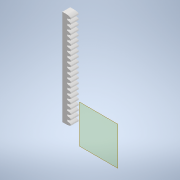
# Autodesk Inventor part: Zahnstange
Saved by Autodesk Inventor 2021 (Build 250183000, 183)
## iProperties
Created: 2021-01-13
Part Number: Zahnstange
Material: Generisch
Document SubType Name: Modeling
Designer: LETPJG
Density: 1 g/cm^3
Appearance: Vorgabe
Author: LETPJG
Autodesk Inventor part; units mm, degrees
ref_plane "YZ Plane" through (0, 0, 0) normal (1, 0, 0) x (0, 1, 0)
ref_plane "XZ Plane" through (0, 0, 0) normal (0, 1, 0) x (-1, 0, 0)
ref_plane "XY Plane" through (0, 0, 0) normal (0, 0, 1) x (1, 0, 0)
ref_plane "Arbeitsebene1" through (0, 0, -5) normal (0, 0, -1) x (-1, 0, 0)
sketch "Skizze1" plane through (0, 0, -5) normal (0, 0, -1) x (-1, 0, 0)
  arc A0 (8.6893, -1.0285) -> (10.9915, -0.4319) centre (7.7825, 7.211) ccw
  arc A1 (10.9915, -0.4319) -> (10.9915, 0.4319) centre (0, 0) ccw
  arc A2 (10.9915, 0.4319) -> (8.6893, 1.0285) centre (7.7825, -7.211) ccw
  line L0 (8.6893, -1.0285) -> (8.6893, 1.0285) construction
  arc A3 (12.6615, 1.2584) -> (14.9637, 0.6618) centre (15.8705, 8.9013) ccw
  arc A4 (12.6615, 2.1221) -> (12.6615, 1.2584) centre (23.6531, 1.6903) ccw
  arc A5 (14.9637, 2.7187) -> (12.6615, 2.1221) centre (15.8705, -5.5208) ccw
  arc A6 (8.6893, 1.0285) -> (8.5819, 1.707) centre (0, 0) ccw construction
  arc A7 (8.6893, 1.0285) -> (8.5819, 1.707) centre (0, 0) ccw construction
  arc A8 (8.6893, 1.0285) -> (8.5819, 1.707) centre (0, 0) ccw construction
  arc A9 (8.6893, 1.0285) -> (8.5819, 1.707) centre (0, 0) ccw construction
  arc A10 (8.6893, 1.0285) -> (8.5819, 1.707) centre (0, 0) ccw construction
  arc A11 (12.6615, 4.1794) -> (14.9637, 3.5828) centre (15.8705, 11.8223) ccw
  arc A12 (12.6615, 5.0431) -> (12.6615, 4.1794) centre (23.6531, 4.6113) ccw
  arc A13 (14.9637, 5.6397) -> (12.6615, 5.0431) centre (15.8705, -2.5998) ccw
  arc A14 (12.6615, 7.1004) -> (14.9637, 6.5038) centre (15.8705, 14.7433) ccw
  arc A15 (12.6615, 7.9641) -> (12.6615, 7.1004) centre (23.6531, 7.5323) ccw
  arc A16 (14.9637, 8.5607) -> (12.6615, 7.9641) centre (15.8705, 0.3212) ccw
  arc A17 (12.6615, 10.0214) -> (14.9637, 9.4248) centre (15.8705, 17.6643) ccw
  arc A18 (12.6615, 10.8851) -> (12.6615, 10.0214) centre (23.6531, 10.4533) ccw
  arc A19 (14.9637, 11.4817) -> (12.6615, 10.8851) centre (15.8705, 3.2422) ccw
  arc A20 (12.6615, 12.9424) -> (14.9637, 12.3458) centre (15.8705, 20.5853) ccw
  arc A21 (12.6615, 13.8061) -> (12.6615, 12.9424) centre (23.6531, 13.3743) ccw
  arc A22 (14.9637, 14.4027) -> (12.6615, 13.8061) centre (15.8705, 6.1632) ccw
  arc A23 (12.6615, 15.8634) -> (14.9637, 15.2668) centre (15.8705, 23.5063) ccw
  arc A24 (12.6615, 16.7271) -> (12.6615, 15.8634) centre (23.6531, 16.2953) ccw
  arc A25 (14.9637, 17.3237) -> (12.6615, 16.7271) centre (15.8705, 9.0842) ccw
  arc A26 (12.6615, 18.7844) -> (14.9637, 18.1878) centre (15.8705, 26.4273) ccw
  arc A27 (12.6615, 19.6481) -> (12.6615, 18.7844) centre (23.6531, 19.2163) ccw
  arc A28 (14.9637, 20.2447) -> (12.6615, 19.6481) centre (15.8705, 12.0052) ccw
  arc A29 (12.6615, 21.7054) -> (14.9637, 21.1088) centre (15.8705, 29.3483) ccw
  arc A30 (12.6615, 22.5691) -> (12.6615, 21.7054) centre (23.6531, 22.1373) ccw
  arc A31 (14.9637, 23.1657) -> (12.6615, 22.5691) centre (15.8705, 14.9262) ccw
  arc A32 (12.6615, 24.6264) -> (14.9637, 24.0298) centre (15.8705, 32.2693) ccw
  arc A33 (12.6615, 25.4901) -> (12.6615, 24.6264) centre (23.6531, 25.0583) ccw
  arc A34 (14.9637, 26.0867) -> (12.6615, 25.4901) centre (15.8705, 17.8472) ccw
  arc A35 (12.6615, 27.5474) -> (14.9637, 26.9508) centre (15.8705, 35.1903) ccw
  arc A36 (12.6615, 28.4111) -> (12.6615, 27.5474) centre (23.6531, 27.9793) ccw
  arc A37 (14.9637, 29.0077) -> (12.6615, 28.4111) centre (15.8705, 20.7682) ccw
  arc A38 (12.6615, 30.4684) -> (14.9637, 29.8718) centre (15.8705, 38.1113) ccw
  arc A39 (12.6615, 31.3321) -> (12.6615, 30.4684) centre (23.6531, 30.9003) ccw
  arc A40 (14.9637, 31.9287) -> (12.6615, 31.3321) centre (15.8705, 23.6892) ccw
  arc A41 (12.6615, 33.3894) -> (14.9637, 32.7928) centre (15.8705, 41.0323) ccw
  arc A42 (12.6615, 34.2531) -> (12.6615, 33.3894) centre (23.6531, 33.8213) ccw
  arc A43 (14.9637, 34.8497) -> (12.6615, 34.2531) centre (15.8705, 26.6102) ccw
  arc A44 (12.6615, 36.3104) -> (14.9637, 35.7138) centre (15.8705, 43.9533) ccw
  arc A45 (12.6615, 37.1741) -> (12.6615, 36.3104) centre (23.6531, 36.7423) ccw
  arc A46 (14.9637, 37.7707) -> (12.6615, 37.1741) centre (15.8705, 29.5312) ccw
  arc A47 (12.6615, 39.2314) -> (14.9637, 38.6348) centre (15.8705, 46.8743) ccw
  arc A48 (12.6615, 40.0951) -> (12.6615, 39.2314) centre (23.6531, 39.6633) ccw
  arc A49 (14.9637, 40.6917) -> (12.6615, 40.0951) centre (15.8705, 32.4522) ccw
  arc A50 (12.6615, 42.1524) -> (14.9637, 41.5558) centre (15.8705, 49.7953) ccw
  arc A51 (12.6615, 43.0161) -> (12.6615, 42.1524) centre (23.6531, 42.5843) ccw
  arc A52 (14.9637, 43.6127) -> (12.6615, 43.0161) centre (15.8705, 35.3732) ccw
  arc A53 (12.6615, 45.0734) -> (14.9637, 44.4768) centre (15.8705, 52.7163) ccw
  arc A54 (12.6615, 45.9371) -> (12.6615, 45.0734) centre (23.6531, 45.5053) ccw
  arc A55 (14.9637, 46.5337) -> (12.6615, 45.9371) centre (15.8705, 38.2942) ccw
  arc A56 (12.6615, 47.9944) -> (14.9637, 47.3978) centre (15.8705, 55.6373) ccw
  arc A57 (12.6615, 48.8581) -> (12.6615, 47.9944) centre (23.6531, 48.4263) ccw
  arc A58 (14.9637, 49.4547) -> (12.6615, 48.8581) centre (15.8705, 41.2152) ccw
  arc A59 (12.6615, 50.9154) -> (14.9637, 50.3188) centre (15.8705, 58.5583) ccw
  arc A60 (12.6615, 51.7791) -> (12.6615, 50.9154) centre (23.6531, 51.3473) ccw
  arc A61 (14.9637, 52.3757) -> (12.6615, 51.7791) centre (15.8705, 44.1362) ccw
  arc A62 (12.6615, 53.8364) -> (14.9637, 53.2398) centre (15.8705, 61.4793) ccw
  arc A63 (12.6615, 54.7001) -> (12.6615, 53.8364) centre (23.6531, 54.2683) ccw
  arc A64 (14.9637, 55.2967) -> (12.6615, 54.7001) centre (15.8705, 47.0572) ccw
  arc A65 (12.6615, 56.7574) -> (14.9637, 56.1608) centre (15.8705, 64.4003) ccw
  arc A66 (12.6615, 57.6211) -> (12.6615, 56.7574) centre (23.6531, 57.1893) ccw
  arc A67 (14.9637, 58.2177) -> (12.6615, 57.6211) centre (15.8705, 49.9782) ccw
  arc A68 (12.6615, 59.6784) -> (14.9637, 59.0818) centre (15.8705, 67.3213) ccw
  arc A69 (12.6615, 60.5421) -> (12.6615, 59.6784) centre (23.6531, 60.1103) ccw
  arc A70 (14.9637, 61.1387) -> (12.6615, 60.5421) centre (15.8705, 52.8992) ccw
  line L1 (14.9637, 61.1387) -> (17.9637, 61.1387)
  line L2 (17.9637, 61.1387) -> (17.9637, 0.6618)
  line L3 (17.9637, 0.6618) -> (14.9637, 0.6618)
  line L4 (14.9637, 2.7187) -> (14.9637, 3.5828)
  line L5 (14.9637, 5.6397) -> (14.9637, 6.5038)
  line L6 (14.9637, 8.5607) -> (14.9637, 9.4248)
  line L7 (14.9637, 11.4817) -> (14.9637, 12.3458)
  line L8 (14.9637, 14.4027) -> (14.9637, 15.2668)
  line L9 (14.9637, 17.3237) -> (14.9637, 18.1878)
  line L10 (14.9637, 20.2447) -> (14.9637, 21.1088)
  line L11 (14.9637, 23.1657) -> (14.9637, 24.0298)
  line L12 (14.9637, 26.0867) -> (14.9637, 26.9508)
  line L13 (14.9637, 29.0077) -> (14.9637, 29.8718)
  line L14 (14.9637, 31.9287) -> (14.9637, 32.7928)
  line L15 (14.9637, 34.8497) -> (14.9637, 35.7138)
  line L16 (14.9637, 37.7707) -> (14.9637, 38.6348)
  line L17 (14.9637, 40.6917) -> (14.9637, 41.5558)
  line L18 (14.9637, 43.6127) -> (14.9637, 44.4768)
  line L19 (14.9637, 46.5337) -> (14.9637, 47.3978)
  line L20 (14.9637, 49.4547) -> (14.9637, 50.3188)
  line L21 (14.9637, 52.3757) -> (14.9637, 53.2398)
  line L22 (14.9637, 55.2967) -> (14.9637, 56.1608)
  line L23 (14.9637, 58.2177) -> (14.9637, 59.0818)
  point P0 (14.9637, 32.3608)
extrude "Extrusion1" add sketch "Skizze1" against normal blind 5
